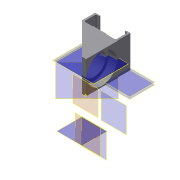
# Autodesk Inventor part: 30_Cube_Insert_Filter_Revolver_Filter_base_single
Saved by Autodesk Inventor 2022 (Build 260153000, 153)
## iProperties
Created: 2021-09-13
Part Number: 30_Cube_Insert_Filter_Revolver_Filter_base_single
Material: Generic
Document SubType Name: Modeling
Designer: diederichbenedict
Density: 1 g/cm^3
Appearance: Default
Mass: 6.97028 g
Surface Area: 48.8121 cm^2
Volume: 6.97028 cm^3
Author: diederichbenedict
Autodesk Inventor part; units mm, degrees
ref_plane "YZ Plane" through (0, 0, 0) normal (1, 0, 0) x (0, 1, 0)
ref_plane "XZ Plane" through (0, 0, 0) normal (0, 1, 0) x (-1, 0, 0)
ref_plane "XY Plane" through (0, 0, 0) normal (0, 0, 1) x (1, 0, 0)
ref_plane "Work Plane1" through (-34.3358, -34.38, 2.0699) normal (0, -1, 0) x (0.7071068, 0, -0.7071068)
ref_plane "Work Plane4" through (-9.5871, -34.38, 28.2329) normal (0, -1, 0) x (1, 0, 0)
ref_plane "Work Plane3" through (-9.5871, -32.38, 28.2329) normal (0, -1, 0) x (1, 0, 0)
sketch "Sketch1" plane through (-9.5871, -34.38, 28.2329) normal (0, -1, 0) x (1, 0, 0)
  line L0 (0.7071, -1.3185) -> (0.7071, -26.3185) construction
  line L1 (0.7071, -1.3185) -> (1.7071, -1.3185) construction
  line L2 (0.7071, -26.3185) -> (1.7071, -26.3185) construction
  line L3 (-4.2929, -0.7071) -> (-31.7929, -28.2071)
  line L4 (-31.7929, -28.2071) -> (0.7071, -28.2071)
  line L5 (0.7071, -28.2071) -> (0.7071, -0.7071)
  line L6 (0.7071, -0.7071) -> (-4.2929, -0.7071)
  line L7 (-4.2929, -0.7071) -> (-4.2929, -28.2071)
  line L8 (-4.2929, -28.2071) -> (0.7071, -28.2071)
  line L9 (0.7071, -0.7071) -> (3.5978, -0.7071)
  line L10 (2.5336, 1.8671) -> (2.3871, 1.8671) projected
  line L11 (0.7071, -0.7071) -> (0.7071, -28.2071)
  line L12 (0.7071, -28.2071) -> (-31.7929, -28.2071)
  point P0 (9.5871, -28.2329)
  dimension "d1" = 5
  dimension "d96" = 27.5
  dimension "d97" = 135
  constraints: 22 end point, 4 perpendicular, 3 horizontal, 2 point on line, 1 collinear, 2 other
  measures "d1" distance of L5.end L3.start
  measures "d96" distance between parallel lines of L4 L6
  measures "d97" angle of L7 L3
extrude "Extrusion1" add sketch "Sketch1" against normal blind 28
ref_plane "Work Plane5" through (-9.5871, -20.38, 28.2329) normal (0, -1, 0) x (1, 0, 0)
ref_plane "Work Plane6" through (-11.0013, -34.38, 27.5258) normal (0, 0, 1) x (1, 0, 0)
sketch "Sketch4" plane through (-8.88, -34.38, 27.5258) normal (-1, 0, 0) x (0, 0, 1)
  line L0 (0, 0) -> (-27.5, 0) projected
  line L1 (-27.5, 28) -> (0, 28) projected
  circle A0 centre (-13.75, 14) radius 10
  line L2 (0, 0) -> (0, 28) projected
  point P0 (-27.5258, 34.38)
  dimension "d89" = 28
  dimension "d90" = 20
  dimension "d91" = 14
  dimension "d98" = 13.75
  constraints: 1 centre point
  measures "d89" distance between parallel lines of L0 L1
  measures "d90" diameter of A0
  measures "d91" distance from line of A0.centre L0
  measures "d98" distance from line of A0.centre L2
extrude "Extrusion4" cut sketch "Sketch4" along normal through all
sketch "Sketch9" plane through (-11.38, -34.38, 30.0258) normal (-0.7071068, 0, 0.7071068) x (0.7071068, 0, 0.7071068)
  ellipse E0 centre (-22.981, 14) end of major axis (-37.1231, 14) minor radius 10 projected
  circle A0 centre (-24.1806, 14) radius 13
  point P0 (-13.1846, 34.38)
  dimension "d129" = 26
  constraints: 1 centre point, 1 other
  measures "d129" diameter of A0
extrude "Extrusion9" cut sketch "Sketch9" against normal blind 3.3 contours E0 A0 | E0 A0 picked at (-17.3557, 13.997) picked at (-25.1272, 3.1067)
sketch "Sketch3" plane through (-8.88, -34.38, 27.5258) normal (-1, 0, 0) x (0, 0, 1)
  circle A0 centre (-13.75, 14) radius 10 projected
  circle A1 centre (-13.75, 14) radius 13
  point P0 (-27.5258, 34.38)
  point P1 (13.1114, 14)
  dimension "d100" = 26
  constraints: 1 centre point, 1 coincident
  measures "d100" diameter of A1
extrude "Extrusion3" cut sketch "Sketch3" along normal blind 8.5 contours A0 | A1
sketch "Sketch13" plane through (-12.38, -34.38, 29.0258) normal (-0.7071068, 0, 0.7071068) x (0.7071068, 0, 0.7071068)
  arc A0 (-7.4246, 14) -> (-7.4246, 14) centre (-21.5668, 14) ccw projected
  circle A1 centre (-7.0668, 25) radius 1.4
  circle A2 centre (-7.0668, 3) radius 1.4
  circle A3 centre (-37.5668, 14) radius 1.4
  point P0 (-11.7703, 34.38)
  point P1 (-18.5424, 14)
  dimension "d101" = 2.8
  dimension "d102" = 2.8
  dimension "d103" = 14.5
  dimension "d104" = 14.5
  dimension "d105" = 16
  dimension "d106" = 2.8
  dimension "d127" = 11
  dimension "d128" = 11
  constraints: 3 centre point, 1 other
  measures "d101" diameter of A2
  measures "d102" diameter of A3
  measures "d103" horizontal distance of A1.centre point (-21.567, 14)
  measures "d104" horizontal distance of point (-21.567, 14) A2.centre
  measures "d105" distance of point (-21.567, 14) A3.centre
  measures "d106" diameter of A1
  measures "d127" vertical distance of A1.centre point (-21.567, 14)
  measures "d128" vertical distance of point (-21.567, 14) A2.centre
extrude "Extrusion13" cut sketch "Sketch13" against normal blind 10 contours A1 | A2 | A3
ref_plane "Arbeitsebene13" through (-3.6065, -62.7242, 27.5258) normal (0, 0, -1) x (-1, 0, 0)
ref_plane "Arbeitsebene16" through (-8.88, -62.38, 27.5258) normal (0, 0, 1) x (1, 0, 0)
sketch "Sketch16" plane through (-8.88, -62.38, 27.5258) normal (0, 0, 1) x (1, 0, 0)
  ellipse E0 centre (-13.3299, 42) end of major axis (-13.3299, 54.75) minor radius 9.0156 projected
  circle A0 centre (-13.3299, 42) radius 1.5708
  point P0 (8.88, 62.38)
  constraints: 1 centre point, 1 coincident, 1 other
extrude "Extrusion15" cut sketch "Sketch16" against normal through all contours A0
ref_plane "Work Plane11" through (-8.88, -20.38, 27.5258) normal (0, -1, 0) x (1, 0, 0)
ref_plane "Arbeitsebene12" through (-8.88, -20.38, 27.5258) normal (0, -1, 0) x (1, 0, 0)
ref_plane "Arbeitsebene15" through (-13.88, -62.38, 0.0258) normal (0, 0, -1) x (1, 0, 0)
sketch "Skizze20" plane through (-13.88, -62.38, 0.0258) normal (0, 0, -1) x (1, 0, 0)
  circle A0 centre (27.7649, 33.0797) radius 1.45
  point P0 (13.88, -62.38)
  dimension "d93" = 2.9
  constraints: 1 centre point
  measures "d93" diameter of A0
extrude "Extrusion17" cut sketch "Skizze20" against normal blind 10
ref_plane "Arbeitsebene14" through (-13.88, -62.38, 27.5258) normal (0, -1, 0) x (1, 0, 0)
sketch "Skizze22" plane through (-13.88, -34.38, 27.5258) normal (0, -1, 0) x (1, 0, 0)
  line L0 (1.0943, -37.15) -> (1.0943, -29.35) projected
  line L1 (1.0943, -29.35) -> (-0.1056, -28.15) projected
  line L2 (-0.1056, -28.15) -> (-24.1056, -28.15) projected
  line L3 (-24.1056, -28.15) -> (-25.3056, -29.35) projected
  line L4 (-25.3056, -29.35) -> (-25.3056, -37.15) projected
  line L5 (-25.3056, -37.15) -> (-24.7056, -37.75) projected
  line L6 (-24.7056, -37.75) -> (-18.1056, -37.75) projected
  line L7 (-18.1056, -37.75) -> (-18.1056, -36.6079) projected
  arc A0 (-17.9505, -36.3766) -> (-18.1056, -36.6079) centre (-17.8556, -36.6079) ccw projected
  arc A1 (-17.9505, -36.3766) -> (-17.3728, -35.8773) centre (-18.4056, -35.2663) ccw projected
  arc A2 (-17.1795, -35.7555) -> (-17.3728, -35.8773) centre (-17.1577, -36.0046) ccw projected
  line L8 (-17.1795, -35.7555) -> (-16.8338, -35.7253) projected
  arc A3 (-16.8338, -35.7253) -> (-16.6056, -35.4762) centre (-16.8556, -35.4762) ccw projected
  line L9 (-16.6056, -35.4762) -> (-16.6056, -35.0238) projected
  arc A4 (-16.6056, -35.0238) -> (-16.8338, -34.7748) centre (-16.8556, -35.0238) ccw projected
  line L10 (-16.8338, -34.7748) -> (-17.2004, -34.7427) projected
  arc A5 (-17.3902, -34.6268) -> (-17.2004, -34.7427) centre (-17.1786, -34.4936) ccw projected
  arc A6 (-17.3902, -34.6268) -> (-17.9505, -34.1559) centre (-18.4056, -35.2663) ccw projected
  arc A7 (-18.1056, -33.9246) -> (-17.9505, -34.1559) centre (-17.8556, -33.9246) ccw projected
  line L11 (-18.1056, -33.9246) -> (-18.1056, -33.25) projected
  line L12 (-18.1056, -33.25) -> (-17.6056, -32.75) projected
  line L13 (-17.6056, -32.75) -> (-6.6057, -32.75) projected
  line L14 (-6.6057, -32.75) -> (-6.1057, -33.25) projected
  line L15 (-6.1057, -33.25) -> (-6.1057, -33.9246) projected
  arc A8 (-6.2608, -34.1559) -> (-6.1057, -33.9246) centre (-6.3557, -33.9246) ccw projected
  arc A9 (-6.2608, -34.1559) -> (-6.8211, -34.6268) centre (-5.8057, -35.2663) ccw projected
  arc A10 (-7.0109, -34.7427) -> (-6.8211, -34.6268) centre (-7.0327, -34.4936) ccw projected
  line L16 (-7.0109, -34.7427) -> (-7.3774, -34.7748) projected
  arc A11 (-7.3774, -34.7748) -> (-7.6057, -35.0238) centre (-7.3557, -35.0238) ccw projected
  line L17 (-7.6057, -35.0238) -> (-7.6057, -35.4762) projected
  arc A12 (-7.6057, -35.4762) -> (-7.3774, -35.7253) centre (-7.3557, -35.4762) ccw projected
  line L18 (-7.3774, -35.7253) -> (-7.0318, -35.7555) projected
  arc A13 (-6.8385, -35.8773) -> (-7.0318, -35.7555) centre (-7.0536, -36.0046) ccw projected
  arc A14 (-6.8385, -35.8773) -> (-6.2608, -36.3766) centre (-5.8057, -35.2663) ccw projected
  arc A15 (-6.1057, -36.6079) -> (-6.2608, -36.3766) centre (-6.3557, -36.6079) ccw projected
  line L19 (-6.1057, -36.6079) -> (-6.1057, -37.75) projected
  line L20 (-6.1057, -37.75) -> (0.4943, -37.75) projected
  line L21 (0.4943, -37.75) -> (1.0943, -37.15) projected
  circle A16 centre (-5.2056, -30.745) radius 2.1 projected
  circle A17 centre (-19.0056, -30.745) radius 2.1 projected
  arc A18 (-17.9505, -36.3766) -> (-17.3728, -35.8773) centre (-18.4056, -35.2662) ccw projected
  arc A19 (-17.1795, -35.7555) -> (-17.3728, -35.8773) centre (-17.1577, -36.0046) ccw projected
  line L22 (-17.1795, -35.7555) -> (-16.8339, -35.7253) projected
  arc A20 (-16.8339, -35.7253) -> (-16.6056, -35.4762) centre (-16.8556, -35.4762) ccw projected
  line L23 (-16.6056, -35.4762) -> (-16.6056, -35.0238) projected
  arc A21 (-16.6056, -35.0238) -> (-16.8339, -34.7747) centre (-16.8556, -35.0238) ccw projected
  line L24 (-16.8339, -34.7747) -> (-17.2004, -34.7427) projected
  arc A22 (-17.3902, -34.6268) -> (-17.2004, -34.7427) centre (-17.1786, -34.4936) ccw projected
  arc A23 (-17.3902, -34.6268) -> (-17.9505, -34.1559) centre (-18.4056, -35.2662) ccw projected
  arc A24 (-18.1056, -33.9246) -> (-17.9505, -34.1559) centre (-17.8556, -33.9246) ccw projected
  line L25 (-18.1056, -33.9246) -> (-18.1056, -33.25) projected
  line L26 (-18.1056, -33.25) -> (-17.6056, -32.75) projected
  line L27 (-17.6056, -32.75) -> (-6.6056, -32.75) projected
  line L28 (-6.6056, -32.75) -> (-6.1056, -33.25) projected
  line L29 (-6.1056, -33.25) -> (-6.1056, -33.9246) projected
  arc A25 (-6.2608, -34.1559) -> (-6.1056, -33.9246) centre (-6.3556, -33.9246) ccw projected
  arc A26 (-6.2608, -34.1559) -> (-6.8211, -34.6268) centre (-5.8057, -35.2662) ccw projected
  arc A27 (-7.0109, -34.7427) -> (-6.8211, -34.6268) centre (-7.0327, -34.4936) ccw projected
  line L30 (-7.0109, -34.7427) -> (-7.3774, -34.7747) projected
  arc A28 (-7.3774, -34.7747) -> (-7.6056, -35.0238) centre (-7.3556, -35.0238) ccw projected
  line L31 (-7.6056, -35.0238) -> (-7.6056, -35.4762) projected
  arc A29 (-7.6056, -35.4762) -> (-7.3774, -35.7253) centre (-7.3556, -35.4762) ccw projected
  line L32 (-7.3774, -35.7253) -> (-7.0318, -35.7555) projected
  arc A30 (-6.8384, -35.8773) -> (-7.0318, -35.7555) centre (-7.0536, -36.0046) ccw projected
  arc A31 (-6.8384, -35.8773) -> (-6.2608, -36.3766) centre (-5.8057, -35.2662) ccw projected
  arc A32 (-6.1056, -36.6079) -> (-6.2608, -36.3766) centre (-6.3556, -36.6079) ccw projected
  line L33 (-6.1056, -36.6079) -> (-6.1056, -37.75) projected
  line L34 (-6.1056, -37.75) -> (0.7943, -37.75) projected
  line L35 (0.7943, -37.75) -> (1.3943, -37.15) projected
  line L36 (1.3943, -37.15) -> (1.3943, -33.75) projected
  arc A33 (1.3943, -32.95) -> (1.3943, -33.75) centre (1.6943, -33.35) ccw projected
  line L37 (1.3943, -32.95) -> (1.3943, -28.35) projected
  line L38 (1.3943, -28.35) -> (0.7943, -27.75) projected
  line L39 (0.7943, -27.75) -> (-5.7056, -27.75) projected
  line L40 (-5.7056, -27.75) -> (-6.1056, -28.15) projected
  line L41 (-6.1056, -28.15) -> (-18.1056, -28.15) projected
  line L42 (-18.1056, -28.15) -> (-18.5056, -27.75) projected
  line L43 (-18.5056, -27.75) -> (-25.0056, -27.75) projected
  line L44 (-25.0056, -27.75) -> (-25.6056, -28.35) projected
  line L45 (-25.6056, -28.35) -> (-25.6056, -37.15) projected
  line L46 (-25.6056, -37.15) -> (-25.0056, -37.75) projected
  line L47 (-25.0056, -37.75) -> (-18.1056, -37.75) projected
  line L48 (-18.1056, -37.75) -> (-18.1056, -36.6079) projected
  arc A34 (-17.9505, -36.3766) -> (-18.1056, -36.6079) centre (-17.8556, -36.6079) ccw projected
  line L49 (-25.0885, -27.55) -> (-18.4228, -27.55)
  line L50 (-18.4228, -27.55) -> (-18.0228, -27.95)
  line L51 (-18.0228, -27.95) -> (-6.1885, -27.95)
  line L52 (-6.1885, -27.95) -> (-5.7885, -27.55)
  line L53 (-5.7885, -27.55) -> (0.8772, -27.55)
  line L54 (0.8772, -27.55) -> (1.5943, -28.2672)
  line L55 (1.5943, -28.2672) -> (1.5943, -33.0672)
  arc A35 (1.5943, -33.0672) -> (1.5943, -33.6329) centre (1.6943, -33.35) ccw
  line L56 (1.5943, -33.6329) -> (1.5943, -37.2329)
  line L57 (1.5943, -37.2329) -> (0.8772, -37.95)
  line L58 (0.8772, -37.95) -> (-6.3056, -37.95)
  line L59 (-6.3056, -37.95) -> (-6.3056, -36.6079)
  arc A36 (-6.3056, -36.6079) -> (-6.3367, -36.5616) centre (-6.3556, -36.6079) ccw
  arc A37 (-7.0106, -35.9791) -> (-6.3367, -36.5616) centre (-5.8057, -35.2662) ccw
  arc A38 (-7.0106, -35.9791) -> (-7.0493, -35.9547) centre (-7.0536, -36.0046) ccw
  line L60 (-7.0493, -35.9547) -> (-7.3949, -35.9245)
  arc A39 (-7.8056, -35.4762) -> (-7.3949, -35.9245) centre (-7.3556, -35.4762) ccw
  line L61 (-7.8056, -35.4762) -> (-7.8056, -35.0238)
  arc A40 (-7.3949, -34.5755) -> (-7.8056, -35.0238) centre (-7.3556, -35.0238) ccw
  line L62 (-7.3949, -34.5755) -> (-7.0283, -34.5434)
  arc A41 (-7.0283, -34.5434) -> (-6.9904, -34.5203) centre (-7.0327, -34.4936) ccw
  arc A42 (-6.3367, -33.9709) -> (-6.9904, -34.5203) centre (-5.8057, -35.2662) ccw
  arc A43 (-6.3367, -33.9709) -> (-6.3056, -33.9246) centre (-6.3556, -33.9246) ccw
  line L63 (-6.3056, -33.9246) -> (-6.3056, -33.3329)
  line L64 (-6.3056, -33.3329) -> (-6.6885, -32.95)
  line L65 (-6.6885, -32.95) -> (-17.5228, -32.95)
  line L66 (-17.5228, -32.95) -> (-17.9056, -33.3329)
  line L67 (-17.9056, -33.3329) -> (-17.9056, -33.9246)
  arc A44 (-17.9056, -33.9246) -> (-17.8746, -33.9709) centre (-17.8556, -33.9246) ccw
  arc A45 (-17.2209, -34.5203) -> (-17.8746, -33.9709) centre (-18.4056, -35.2662) ccw
  arc A46 (-17.2209, -34.5203) -> (-17.183, -34.5434) centre (-17.1786, -34.4936) ccw
  line L68 (-17.183, -34.5434) -> (-16.8164, -34.5755)
  arc A47 (-16.4056, -35.0238) -> (-16.8164, -34.5755) centre (-16.8556, -35.0238) ccw
  line L69 (-16.4056, -35.0238) -> (-16.4056, -35.4762)
  arc A48 (-16.8164, -35.9245) -> (-16.4056, -35.4762) centre (-16.8556, -35.4762) ccw
  line L70 (-16.8164, -35.9245) -> (-17.162, -35.9547)
  arc A49 (-17.162, -35.9547) -> (-17.2007, -35.9791) centre (-17.1577, -36.0046) ccw
  arc A50 (-17.8746, -36.5616) -> (-17.2007, -35.9791) centre (-18.4056, -35.2662) ccw
  arc A51 (-17.8746, -36.5616) -> (-17.9056, -36.6079) centre (-17.8556, -36.6079) ccw
  line L71 (-17.9056, -36.6079) -> (-17.9056, -37.95)
  line L72 (-17.9056, -37.95) -> (-25.0885, -37.95)
  line L73 (-25.0885, -37.95) -> (-25.8056, -37.2329)
  line L74 (-25.8056, -37.2329) -> (-25.8056, -28.2672)
  line L75 (-25.8056, -28.2672) -> (-25.0885, -27.55)
  line L76 (-27.5, -27.5) -> (5, -27.5) projected
  line L77 (-27.5, -27.5) -> (-27.5, -38.95)
  line L78 (-27.5, -38.95) -> (-23.1356, -38.95)
  line L79 (-23.1356, -38.95) -> (-23.1356, -37.95)
  line L80 (-0.5269, -37.95) -> (-0.5269, -38.95)
  line L81 (-0.5269, -38.95) -> (3.0943, -38.95)
  line L82 (3.0943, -38.95) -> (3.0943, -27.5)
  point P0 (13.88, -27.5258)
  point P1 (-24.0858, -24.0858)
  dimension "d123" = 0.2
  dimension "d124" = 1
  dimension "d125" = 1
  dimension "d126" = 1.5
  constraints: 66 end point, 34 point on circle, 17 centre point, 5 perpendicular, 3 point on line, 1 vertical, 43 other
  measures "d123" distance between parallel lines of L43 L49
  measures "d124" distance between parallel lines of L72 L78
  measures "d125" distance between parallel lines of L58 L81
  measures "d126" distance between parallel lines of L55 L82
extrude "Extrusion18" add sketch "Skizze22" against normal up to surface (28 mm away) contours L75 L74 L73 L72 L79 L78 L77 L76 L82 L81 L80 L58 L57 L56 A35 L55 L54 L53 L52 L51 L50 L49
ref_plane "Arbeitsebene17" through (-13.88, -62.38, 27.5258) normal (0, -1, 0) x (1, 0, 0)
sketch "Skizze23" plane through (-13.88, -62.38, 27.5258) normal (0, -1, 0) x (1, 0, 0)
  line L0 (5, -27.5) -> (5, 0) projected
  line L1 (5, 0) -> (0, 0) projected
  line L2 (0, 0) -> (-27.5, -27.5) projected
  line L3 (3, -39.05) -> (5, -37.05) projected
  line L4 (5.8412, 1.6556) -> (3.5, 1.6556)
  line L5 (3.5, 1.6556) -> (3.5, -38.55)
  line L6 (3.5, -38.55) -> (5.8412, -38.55)
  line L7 (5.8412, -38.55) -> (5.8412, 1.6556)
  line L8 (3.0943, -27.5) -> (5, -27.5) projected
  line L9 (-27.5, -27.5) -> (-27.5, -37.45) projected
  line L10 (-26, -38.95) -> (-23.1356, -38.95) projected
  line L11 (-23.1356, -38.95) -> (-23.1356, -37.95) projected
  line L12 (-23.1356, -37.95) -> (-25.0885, -37.95) projected
  line L13 (-25.0885, -37.95) -> (-25.8056, -37.2329) projected
  line L14 (-25.8056, -37.2329) -> (-25.8056, -28.2672) projected
  line L15 (-25.8056, -28.2672) -> (-25.0885, -27.55) projected
  line L16 (-25.0885, -27.55) -> (-18.4228, -27.55) projected
  line L17 (-18.4228, -27.55) -> (-18.0228, -27.95) projected
  line L18 (-18.0228, -27.95) -> (-6.1885, -27.95) projected
  line L19 (-6.1885, -27.95) -> (-5.7885, -27.55) projected
  line L20 (-5.7885, -27.55) -> (0.8772, -27.55) projected
  line L21 (0.8772, -27.55) -> (1.5943, -28.2672) projected
  line L22 (1.5943, -28.2672) -> (1.5943, -33.0672) projected
  arc A0 (1.5943, -33.0672) -> (1.5943, -33.6329) centre (1.6943, -33.35) ccw projected
  line L23 (1.5943, -33.6329) -> (1.5943, -37.2329) projected
  line L24 (1.5943, -37.2329) -> (0.8772, -37.95) projected
  line L25 (0.8772, -37.95) -> (-0.5269, -37.95) projected
  line L26 (-0.5269, -37.95) -> (-0.5269, -38.95) projected
  line L27 (-0.5269, -38.95) -> (1.5943, -38.95) projected
  line L28 (3.0943, -37.45) -> (3.0943, -27.5) projected
  line L29 (3.0943, -37.45) -> (1.5943, -38.95) projected
  line L30 (-26, -38.95) -> (-27.5, -37.45) projected
  point P0 (13.88, -27.5258)
  constraints: 8 end point, 2 parallel, 1 horizontal, 1 perpendicular, 1 point on line
extrude "Extrusion19" cut sketch "Skizze23" against normal through all contours L8 L5 L1 L0 | L0 L1 L5 L4 L7 L6 L8
ref_plane "Work Plane2" through (41.82, -7.88, -4) normal (0, -1, 0) x (1, 0, 0)
equation "\"d91\" = 0.5 * d89"
equation "\"d98\" = 0.5 * d96"
body "Solid1"
